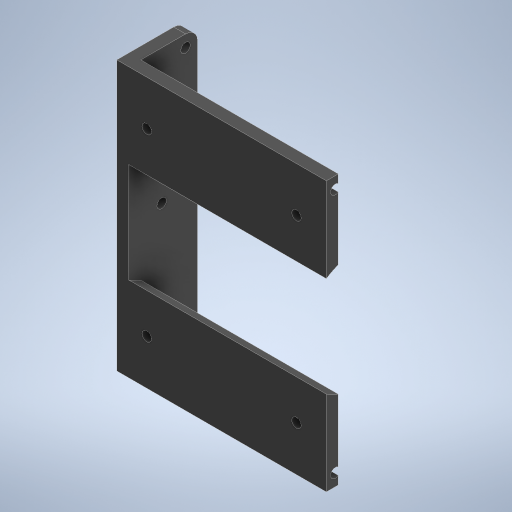
# Autodesk Inventor part: bluetooth_setter
Saved by Autodesk Inventor 2024.1 (Build 281209000, 209)
## iProperties
Created: 2024-02-15
Part Number: bluetooth_setter
Material: 一般
Document SubType Name: Modeling
Designer: hibik
Density: 1 g/cm^3
Appearance: 既定
Author: hibik
Autodesk Inventor part; units mm, degrees
ref_plane "YZ Plane" through (0, 0, 0) normal (1, 0, 0) x (0, 1, 0)
ref_plane "XZ Plane" through (0, 0, 0) normal (0, 1, 0) x (-1, 0, 0)
ref_plane "XY Plane" through (0, 0, 0) normal (0, 0, 1) x (1, 0, 0)
sketch "スケッチ1" plane through (0, 0, 0) normal (1, 0, 0) x (0, 1, 0)
  line L0 (45, 0) -> (0, 0)
  line L1 (0, 0) -> (0, -11.5)
  line L2 (0, -11.5) -> (45, -11.5)
  line L3 (45, -11.5) -> (45, 0)
  dimension "d0" = 45
  dimension "d1" = 11.5
  constraints: 8 end point, 2 parallel, 1 coincident, 1 horizontal, 1 perpendicular
  measures "d0" distance of L0.start L0.end
  measures "d1" distance of L2.end L0.start
extrude "押し出し1" add sketch "スケッチ1" along normal blind 2
sketch "スケッチ2" plane through (2, 0, 0) normal (1, 0, 0) x (0, 0, -1)
  circle A0 centre (1.5, 43) radius 0.8 projected
  circle A1 centre (9.4807, 43) radius 0.8 projected
  circle A2 centre (9.5, 2) radius 0.8 projected
  circle A3 centre (1.5, 2) radius 0.8 projected
  circle A4 centre (5.5, 22.5) radius 0.8 projected
  point P0 (0, 0)
extrude "押し出し2" cut sketch "スケッチ2" against normal through all
fillet "フィレット1" radius 2 2 edges at (1, 45, -11.5) (1, 0, -11.5)
sketch "スケッチ3" plane through (0, 0, 0) normal (-1, 0, 0) x (0, 0, 1)
  circle A0 centre (-5.5, 22.5) radius 0.8 projected
  circle A1 centre (-5.5, 22.5) radius 10
  line L0 (-2, 45) -> (0, 45)
  line L1 (0, 45) -> (0, 0)
  line L2 (0, 0) -> (-2, 0)
  line L3 (-2, 0) -> (-2, 45)
  line L4 (-9.5, 45) -> (0, 45) projected
  line L5 (0, 0) -> (-9.5, 0) projected
  circle A2 centre (-5.5, 22.5) radius 0.8 projected
  arc A3 (-11.5, 2) -> (-9.5, 0) centre (-9.5, 2) ccw projected
  line L6 (0, 0) -> (-9.5, 0) projected
  line L7 (0, 45) -> (0, 0) projected
  line L8 (-9.5, 45) -> (0, 45) projected
  arc A4 (-9.5, 45) -> (-11.5, 43) centre (-9.5, 43) ccw projected
  line L9 (-11.5, 2) -> (-11.5, 43) projected
  circle A5 centre (-1.5, 43) radius 0.8 projected
  circle A6 centre (-1.5, 2) radius 0.8 projected
  point P0 (-2, 31.8675)
  point P1 (-2, 13.1325)
  point P2 (0, 14.1484)
  point P3 (0, 30.8516)
  point P4 (-11.5, 14.5)
  point P5 (-11.5, 30.5)
  point P6 (-2, 45)
  point P7 (-2, 43.6245)
  point P8 (-2, 42.3755)
  point P9 (-2, 2.6245)
  point P10 (-2, 1.3755)
  dimension "d7" = 20
  dimension "d34" = 2
  constraints: 8 end point, 2 collinear, 2 parallel, 1 centre point, 1 coincident, 1 horizontal, 1 perpendicular
  measures "d7" diameter of A1
  measures "d34" distance between parallel lines of L1 L3
extrude "押し出し3" add sketch "スケッチ3" against normal blind 35 contours A1 L3 A5 L0 L1 | L1 L2 L3 A6 A1
sketch "スケッチ6" plane through (0, 0, 0) normal (0, 0, 1) x (1, 0, 0)
  line L0 (5, 37.5) -> (30, 37.5) construction
  line L1 (30, 37.5) -> (30, 7.5) construction
  line L2 (30, 7.5) -> (5, 7.5) construction
  line L3 (5, 7.5) -> (5, 37.5) construction
  line L4 (0, 45) -> (35, 45) projected
  line L5 (0, 0) -> (35, 0) projected
  line L6 (35, 45) -> (35, 30.8516) projected
  line L7 (0, 45) -> (0, 0) projected
  circle A0 centre (5, 37.5) radius 0.8
  circle A1 centre (30, 37.5) radius 0.8
  circle A2 centre (5, 7.5) radius 0.8
  circle A3 centre (30, 7.5) radius 0.8
  dimension "d35" = 25
  dimension "d36" = 30
  dimension "d37" = 7.5
  dimension "d38" = 7.5
  dimension "d39" = 5
  dimension "d40" = 5
  dimension "d41" = 1.6
  dimension "d42" = 1.6
  dimension "d43" = 1.6
  dimension "d44" = 1.6
  constraints: 8 end point, 4 centre point, 4 coincident, 2 parallel, 1 horizontal, 1 perpendicular
  measures "d35" distance of L1.end L2.end
  measures "d36" distance of L0.end L1.end
  measures "d37" distance between parallel lines of L4 L0
  measures "d38" distance between parallel lines of L5 L2
  measures "d39" distance between parallel lines of L6 L1
  measures "d40" distance between parallel lines of L7 L3
  measures "d41" diameter of A0
  measures "d42" diameter of A1
  measures "d43" diameter of A2
  measures "d44" diameter of A3
extrude "押し出し6" cut sketch "スケッチ6" against normal through all
equation "\"d37\" = d38"
equation "\"d39\" = d40"
